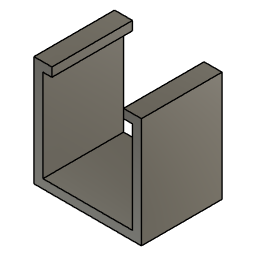
clamp (Autodesk Fusion 360 design; units mm, degrees)
Autodesk Fusion 360 part; units mm, degrees
sketch "Sketch1" plane through (0, 0, 0) normal (0, 0, 1) x (1, 0, 0)
  line L0 (10, 9) -> (-10, 9)
  line L1 (-10, 9) -> (-10, -9)
  line L2 (-10, -9) -> (10, -9)
  line L3 (10, -9) -> (10, 9)
  line L4 (10, 9) -> (-10, -9) construction
  line L5 (-10, 9) -> (10, -9) construction
  line L6 (10, 9) -> (12, 9)
  line L7 (12, 9) -> (12, -9)
  line L8 (12, -9) -> (10, -9)
  line L9 (10, -9) -> (10, 9)
  line L10 (-10, 9) -> (-12, 9)
  line L11 (-12, 9) -> (-12, -9)
  line L12 (-12, -9) -> (-10, -9)
  line L13 (-10, -9) -> (-10, 9)
  dimension "d1" = 20
  dimension "d2" = 18
  dimension "d3" = 2
  constraint horizontal L0
  constraint perpendicular L0 L1
  constraint parallel L0 L2
  constraint parallel L1 L3
  constraint coincident L4 origin
  constraint coincident L5 origin
  constraint horizontal L6
  constraint vertical L7
  constraint horizontal L8
  constraint vertical L9
  constraint horizontal L10
  constraint vertical L11
  constraint horizontal L12
  constraint vertical L13
  measures "d1" distance of L1.end L2.end
  measures "d2" distance of L0.end L1.end
  measures "d3" distance of L0.end L10.end
extrude "Extrude1" add sketch "Sketch1" along normal blind 2 contours L0 L1 L2 L3 L9 L13
extrude "Extrude2" add sketch "Sketch1" along normal blind 22.6 contours L3 L6 L7 L8 L9 | L1 L10 L11 L12 L13
sketch "Sketch2" plane through (0, -9, 0) normal (0, -1, 0) x (1, 0, 0)
  line L0 (-12, 0) -> (12, 0)
  line L1 (12, 0) -> (12, 22.6)
  line L2 (12, 22.6) -> (10, 22.6)
  line L3 (10, 22.6) -> (10, 2)
  line L4 (10, 2) -> (-10, 2)
  line L5 (-10, 2) -> (-10, 22.6)
  line L6 (-10, 22.6) -> (-12, 22.6)
  line L7 (-12, 22.6) -> (-12, 0)
  line L8 (-12, 22.6) -> (-8, 22.6)
  line L9 (-8, 22.6) -> (-8, 24.6)
  line L10 (-8, 24.6) -> (-12, 24.6)
  line L11 (-12, 24.6) -> (-12, 22.6)
  line L12 (12, 22.6) -> (8, 22.6)
  line L13 (8, 22.6) -> (8, 24.6)
  line L14 (8, 24.6) -> (12, 24.6)
  line L15 (12, 24.6) -> (12, 22.6)
  dimension "d8" = 4
  dimension "d9" = 2
  dimension "d10" = 4
  dimension "d11" = 2
  constraint horizontal L8
  constraint vertical L9
  constraint horizontal L10
  constraint vertical L11
  constraint coincident L6.end L7.start
  constraint horizontal L12
  constraint vertical L13
  constraint horizontal L14
  constraint vertical L15
  constraint coincident L1.end L2.start
  measures "d8" distance of L6.end L8.end
  measures "d9" distance of L6.end L10.end
  measures "d10" distance of L1.end L12.end
  measures "d11" distance of L1.end L14.end
extrude "Extrude3" add sketch "Sketch2" against normal blind 18 contours L6 L8 L9 L10 L11 | L2 L12 L13 L14 L15
